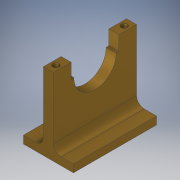
# Autodesk Inventor part: Part8
Saved by Autodesk Inventor 2019 (Build 230136000, 136)
## iProperties
Created: 2022-01-28
Part Number: Part8
Material: Generic
Document SubType Name: Modeling
Designer: Sepehr
Density: 1 g/cm^3
Appearance: Default
Author: Sepehr
Autodesk Inventor part; units mm, degrees
ref_plane "YZ Plane" through (0, 0, 0) normal (1, 0, 0) x (0, 1, 0)
ref_plane "XZ Plane" through (0, 0, 0) normal (0, 1, 0) x (-1, 0, 0)
ref_plane "XY Plane" through (0, 0, 0) normal (0, 0, 1) x (1, 0, 0)
sketch "Sketch1" plane through (0, 0, 0) normal (0, 1, 0) x (-1, 0, 0)
  line L0 (-2250, 2700) -> (2250, 2700)
  line L1 (2250, -2700) -> (-2250, -2700)
  line L2 (-2250, -2700) -> (-2250, 2700)
  line L3 (1300, -1375) -> (1300, -1550)
  line L4 (1300, -1550) -> (2250, -1550)
  line L5 (1300, 1375) -> (1300, 1550)
  line L6 (1300, 1550) -> (2250, 1550)
  arc A0 (1300, 1375) -> (1300, -1375) centre (1300, 0) ccw
  line L7 (2250, 2700) -> (2250, 1550)
  line L8 (2250, -1550) -> (2250, -2700)
  constraints: 18 end point, 6 perpendicular, 3 parallel, 2 point on circle, 2 vertical, 1 centre point, 1 horizontal
extrude "Extrusion1" add sketch "Sketch1" along normal mid plane 650
sketch "Sketch2" plane through (2250, -325, -2700) normal (1, 0, 0) x (0, 0, -1)
  line L0 (-5400, 1950) -> (0, 1950)
  line L1 (0, 1950) -> (0, -1300)
  line L2 (0, -1300) -> (-5400, -1300)
  line L3 (-5400, -1300) -> (-5400, 1950)
  line L4 (-5400, 1950) -> (0, -1300) construction
  line L5 (0, 1950) -> (-5400, -1300) construction
  point P0 (-2700, 325)
  dimension "d10" = 3250
  constraints: 12 end point, 2 midpoint, 2 parallel, 1 horizontal, 1 perpendicular
  measures "d10" distance of L0.end L1.end
extrude "Extrusion2" add sketch "Sketch2" along normal blind 500
fillet "Fillet1" radius 500 2 edges at (2250, 325, 0) (2250, -325, 0)
sketch "Sketch3" plane through (-2250, -325, 2700) normal (-1, 0, 0) x (0, 0, 1)
  line L0 (0, 0) -> (-5400, 0) projected
  line L1 (0, 0) -> (0, 325)
  line L2 (0, 1950) -> (0, -1300) projected
  line L3 (0, 325) -> (-481.017, 325)
  circle A0 centre (-481.017, 325) radius 200
  line L4 (-5400, 0) -> (-5400, 325)
  line L5 (-5400, -1300) -> (-5400, 1950) projected
  line L6 (-5400, 325) -> (-4918.983, 325)
  circle A1 centre (-4918.983, 325) radius 200
  point P0 (-2700, 325)
  dimension "d14" = 325
  dimension "d15" = 481.017
  dimension "d16" = 400
  dimension "d17" = 325
  dimension "d18" = 481.017
  dimension "d19" = 400
  constraints: 8 end point, 2 centre point, 2 coincident, 2 midpoint, 2 perpendicular
  measures "d14" distance of L0.start L1.end
  measures "d15" distance of L1.end L3.end
  measures "d16" diameter of A0
  measures "d17" distance of L0.end L4.end
  measures "d18" distance of L4.end L6.end
  measures "d19" diameter of A1
extrude "Extrusion3" cut sketch "Sketch3" against normal blind 1100
body "Solid1"
